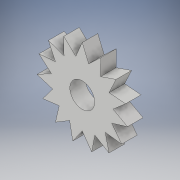
# Autodesk Inventor part: Backdrop Gear 2
Saved by Autodesk Inventor 2018 (Build 220112000, 112)
## iProperties
Created: 2018-12-13
Part Number: Backdrop Gear 2
Material: Generic
Document SubType Name: Modeling
Designer: F8PLTW
Density: 1 g/cm^3
Appearance: Default
Author: F8PLTW
Autodesk Inventor part; units mm, degrees
ref_plane "YZ Plane" through (0, 0, 0) normal (1, 0, 0) x (0, 1, 0)
ref_plane "XZ Plane" through (0, 0, 0) normal (0, 1, 0) x (-1, 0, 0)
ref_plane "XY Plane" through (0, 0, 0) normal (0, 0, 1) x (1, 0, 0)
sketch "Sketch1" plane through (0, 0, 0) normal (0, 0, 1) x (1, 0, 0)
  line L0 (0, 5.85) -> (1.4732, 5.85)
  line L1 (1.4732, 5.85) -> (-1.4732, 5.85)
  line L2 (-1.4732, 5.85) -> (0, 9.3136)
  line L3 (0, 9.3136) -> (1.4732, 5.85)
  line L4 (-3.7252, 4.745) -> (-3.7882, 8.5084)
  line L5 (-3.7882, 8.5084) -> (-1.0336, 5.9434)
  line L6 (-1.0336, 5.9434) -> (-3.7252, 4.745)
  line L7 (-5.3332, 2.8196) -> (-6.9213, 6.232)
  line L8 (-6.9213, 6.232) -> (-3.3616, 5.0092)
  line L9 (-3.3616, 5.0092) -> (-5.3332, 2.8196)
  line L10 (-6.0189, 0.4067) -> (-8.8578, 2.8781)
  line L11 (-8.8578, 2.8781) -> (-5.1084, 3.2088)
  line L12 (-5.1084, 3.2088) -> (-6.0189, 0.4067)
  line L13 (-5.664, -2.0766) -> (-9.2626, -0.9735)
  line L14 (-9.2626, -0.9735) -> (-5.9719, 0.8536)
  line L15 (-5.9719, 0.8536) -> (-5.664, -2.0766)
  line L16 (-4.3296, -4.2008) -> (-8.0658, -4.6568)
  line L17 (-8.0658, -4.6568) -> (-5.8028, -1.6492)
  line L18 (-5.8028, -1.6492) -> (-4.3296, -4.2008)
  line L19 (-2.2467, -5.5987) -> (-5.4744, -7.5349)
  line L20 (-5.4744, -7.5349) -> (-4.6304, -3.8668)
  line L21 (-4.6304, -3.8668) -> (-2.2467, -5.5987)
  line L22 (0.2247, -6.0285) -> (-1.9364, -9.1101)
  line L23 (-1.9364, -9.1101) -> (-2.6573, -5.4159)
  line L24 (-2.6573, -5.4159) -> (0.2247, -6.0285)
  line L25 (2.6573, -5.4159) -> (1.9364, -9.1101)
  line L26 (1.9364, -9.1101) -> (-0.2247, -6.0285)
  line L27 (-0.2247, -6.0285) -> (2.6573, -5.4159)
  line L28 (4.6304, -3.8668) -> (5.4744, -7.5349)
  line L29 (5.4744, -7.5349) -> (2.2467, -5.5987)
  line L30 (2.2467, -5.5987) -> (4.6304, -3.8668)
  line L31 (5.8028, -1.6492) -> (8.0658, -4.6568)
  line L32 (8.0658, -4.6568) -> (4.3296, -4.2008)
  line L33 (4.3296, -4.2008) -> (5.8028, -1.6492)
  line L34 (5.9719, 0.8536) -> (9.2626, -0.9735)
  line L35 (9.2626, -0.9735) -> (5.664, -2.0766)
  line L36 (5.664, -2.0766) -> (5.9719, 0.8536)
  line L37 (5.1084, 3.2088) -> (8.8578, 2.8781)
  line L38 (8.8578, 2.8781) -> (6.0189, 0.4067)
  line L39 (6.0189, 0.4067) -> (5.1084, 3.2088)
  line L40 (3.3616, 5.0092) -> (6.9213, 6.232)
  line L41 (6.9213, 6.232) -> (5.3332, 2.8196)
  line L42 (5.3332, 2.8196) -> (3.3616, 5.0092)
  line L43 (1.0336, 5.9434) -> (3.7882, 8.5084)
  line L44 (3.7882, 8.5084) -> (3.7252, 4.745)
  line L45 (3.7252, 4.745) -> (1.0336, 5.9434)
  circle A0 centre (0, 0) radius 6.0326
  dimension "d6" = 1.4732
  dimension "d7" = 2.9464
  dimension "d10" = 360
  constraints: 92 end point, 1 coincident, 1 point on line, 94 other
  measures "d6" distance of L0.start L0.end
  measures "d7" distance of L0.end L1.end
extrude "Extrusion1" add sketch "Sketch1" along normal blind 3.175
sketch "Sketch2" plane through (0, 0, 3.175) normal (0, 0, 1) x (1, 0, 0)
  circle A0 centre (0, 0) radius 2.54
  dimension "d14" = 5.08
  constraints: 1 centre point, 1 coincident
  measures "d14" diameter of A0
extrude "Extrusion2" cut sketch "Sketch2" against normal blind 3.175
body "Solid1"
